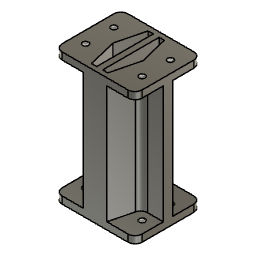
0812_arm_short v2 (Autodesk Fusion 360 design; units mm, degrees)
Autodesk Fusion 360 part; units mm, degrees
sketch "스케치1" plane through (0, 0, 0) normal (0, 0, 1) x (1, 0, 0)
  line L0 (-17, 14) -> (17, 14)
  line L1 (17, 14) -> (17, -14)
  line L2 (17, -14) -> (-17, -14)
  line L3 (-17, -14) -> (-17, 14)
  line L4 (0, 14) -> (0, -14) construction
  line L5 (-12, 6) -> (12, 6) construction
  line L6 (12, 6) -> (12, -6) construction
  line L7 (12, -6) -> (-12, -6) construction
  line L8 (-12, -6) -> (-12, 6) construction
  line L9 (0, 6) -> (0, -6) construction
  circle A0 centre (-12, 6) radius 1.5
  circle A1 centre (12, 6) radius 1.5
  circle A2 centre (-12, -6) radius 1.5
  circle A3 centre (12, -6) radius 1.5
  line L10 (-5, 14) -> (5, 14)
  line L11 (5, 14) -> (5, -14) construction
  line L12 (5, -14) -> (-5, -14)
  line L13 (-5, -14) -> (-5, 14) construction
  line L14 (-17, 2) -> (17, 2) construction
  line L15 (17, 2) -> (17, -2)
  line L16 (17, -2) -> (-17, -2) construction
  line L17 (-17, -2) -> (-17, 2)
  line L18 (0, 2) -> (0, -2) construction
  line L19 (0, 14) -> (0, -14) construction
  line L20 (-5, 14) -> (-8, 2)
  line L21 (5, 14) -> (8, 2)
  line L22 (-8, -2) -> (-5, -14)
  line L23 (8, -2) -> (5, -14)
  line L24 (-17, 2) -> (-8, 2)
  line L25 (8, 2) -> (17, 2)
  line L26 (8, -2) -> (17, -2)
  line L27 (-17, -2) -> (-8, -2)
  line L28 (-3.4384, 12) -> (3.4384, 12)
  line L29 (3.4384, 12) -> (6.4384, 0)
  line L30 (6.4384, 0) -> (3.4384, -12)
  line L31 (3.4384, -12) -> (-3.4384, -12)
  line L32 (-3.4384, -12) -> (-6.4384, 0)
  line L33 (-6.4384, 0) -> (-3.4384, 12)
  line L34 (0, 12) -> (0, -12) construction
  line L35 (-6.4384, 0) -> (6.4384, 0) construction
  line L36 (-1.25, 14) -> (1.25, 14)
  line L37 (1.25, 14) -> (1.25, -14)
  line L38 (1.25, -14) -> (-1.25, -14)
  line L39 (-1.25, -14) -> (-1.25, 14)
  line L40 (0, 14) -> (0, -14) construction
  point P0 (0, 14)
  point P1 (0, -14)
  point P2 (0, 6)
  point P3 (0, -6)
  point P4 (0, 2)
  point P5 (0, -2)
  point P6 (0, 14)
  point P7 (0, -14)
  point P8 (-8, 2)
  point P9 (-8, -2)
  point P10 (8, 2)
  point P11 (8, -2)
  point P12 (-17, 2)
  point P13 (-17, -2)
  point P14 (17, -2)
  point P15 (17, 2)
  point P16 (0, 12)
  point P17 (0, -12)
  point P18 (0, 14)
  point P19 (0, -14)
  point P20 (-1.25, 12)
  point P21 (-1.25, 12)
  point P22 (1.25, 12)
  point P23 (1.25, 12)
  point P24 (-1.25, -12)
  point P25 (-1.25, -12)
  point P26 (1.25, -12)
  point P27 (1.25, -12)
  dimension "d1" = 34
  dimension "d2" = 28
  dimension "d3" = 24
  dimension "d4" = 12
  dimension "d5" = 3
  dimension "d6" = 3
  dimension "d7" = 3
  dimension "d8" = 3
  dimension "d11" = 10
  dimension "d12" = 28
  dimension "d13" = 34
  dimension "d14" = 4
  dimension "d15" = 9
  dimension "d16" = 9
  dimension "d17" = 9
  dimension "d18" = 9
  dimension "d19" = 2
  dimension "d20" = 2
  dimension "d21" = 2
  dimension "d22" = 2.5
  dimension "d23" = 28
  constraint horizontal L0
  constraint vertical L1
  constraint horizontal L2
  constraint vertical L3
  constraint midpoint L0 P18
  constraint midpoint L2 P19
  constraint coincident P18 P6
  constraint coincident P19 P7
  constraint midpoint L4 origin
  constraint horizontal L5
  constraint vertical L6
  constraint horizontal L7
  constraint vertical L8
  constraint midpoint L5 P2
  constraint midpoint L7 P3
  constraint coincident P2 L9.start
  constraint coincident P3 L9.end
  constraint midpoint L9 origin
  constraint coincident L5.start L8.end
  constraint coincident L5.end L6.start
  constraint coincident L7.end L8.start
  constraint coincident L6.end L7.start
  constraint horizontal L10
  constraint vertical L11
  constraint horizontal L12
  constraint vertical L13
  constraint horizontal L14
  constraint vertical L15
  constraint horizontal L16
  constraint vertical L17
  constraint midpoint L14 P4
  constraint midpoint L16 P5
  constraint coincident P4 L18.start
  constraint coincident P5 L18.end
  constraint midpoint L18 origin
  constraint midpoint L10 P18
  constraint midpoint L12 P19
  constraint midpoint L19 origin
  constraint coincident L14 P8
  constraint coincident L16 P9
  constraint coincident L14 P10
  constraint coincident L16 P11
  constraint coincident P12 L14.start
  constraint coincident P13 L16.end
  constraint coincident P14 L15.end
  constraint coincident P15 L14.end
  constraint coincident P8 L20.end
  constraint coincident P10 L21.end
  constraint coincident P9 L22.start
  constraint coincident P11 L23.start
  constraint horizontal L28
  constraint parallel L28 L31
  constraint midpoint L28 P16
  constraint midpoint L31 P17
  constraint coincident P16 L34.start
  constraint coincident P17 L34.end
  constraint midpoint L34 origin
  constraint perpendicular L28 L34
  constraint coincident L29 L30.start
  constraint midpoint L35 origin
  constraint perpendicular L34 L35
  constraint parallel L21 L29
  constraint parallel L23 L30
  constraint horizontal L36
  constraint vertical L37
  constraint horizontal L38
  constraint vertical L39
  constraint midpoint L36 P18
  constraint midpoint L38 P19
  constraint midpoint L40 origin
  constraint coincident L28 P21
  constraint coincident L39 P21
  constraint coincident P21 P20
  constraint coincident L28 P23
  constraint coincident L37 P23
  constraint coincident P23 P22
  constraint coincident L31 P25
  constraint coincident L39 P25
  constraint coincident L31 P27
  constraint coincident L37 P27
  constraint coincident P25 P24
  constraint coincident P27 P26
  measures "d1" distance of L0.start L0.end
  measures "d2" distance of L0.start L2.end
  measures "d3" distance of L5.start L5.end
  measures "d4" distance of L5.start L7.end
  measures "d5" diameter of A0
  measures "d6" diameter of A1
  measures "d7" diameter of A2
  measures "d8" diameter of A3
  measures "d11" distance of L10.start L10.end
  measures "d12" distance of L10.start L12.end
  measures "d13" distance of P12 P15
  measures "d14" distance of P12 P13
  measures "d15" distance of P8 P12
  measures "d16" distance of P9 P13
  measures "d17" distance of P10 P15
  measures "d18" distance of P11 P14
  measures "d19" distance of L10 L28
  measures "d20" distance of L21 L29
  measures "d21" distance of L23 L30
  measures "d22" distance of L36.start L36.end
  measures "d23" distance of L36.start L38.end
extrude "돌출2" add sketch "스케치1" along normal blind 56 contours L0 L2 L3 L10 L12 L17 L20 L22 L24 L27 L28 L31 L32 L33 L39 | L0 L10 L28 L36 L37 L39 | L0 L1 L2 L10 L12 L15 L21 L23 L25 L26 L28 L29 L30 L31 L37 | L28 L31 L37 L39 | L2 L12 L31 L37 L38 L39
extrude "돌출3" add sketch "스케치1" along normal blind 3 contours L0 L3 L20 L24 | L2 L3 L22 L27 | L0 L1 L21 L25 | L1 L2 L23 L26
extrude "돌출4" add sketch "스케치1" along normal blind 3 from surface at 53 contours L0 L3 L20 L24 | L2 L3 L22 L27 | L0 L1 L21 L25 | L1 L2 L23 L26
extrude "돌출5" add sketch "스케치1" along normal blind 3 contours L28 L31 L32 L33 L39 | L28 L29 L30 L31 L37
thread "스레드1" "ISO Metric profile 3.0 M3x0.5 6H" major diameter 3.086 minor diameter 2.529 pitch 0.5 angle 60 resizes the face on face at (-10.5019, 5.9252, 55)
thread "스레드2" "ISO Metric profile 3.0 M3x0.5 6H" major diameter 3.086 minor diameter 2.529 pitch 0.5 angle 60 resizes the face on face at (-10.5019, -6.0748, 55)
thread "스레드3" "ISO Metric profile 3.0 M3x0.5 6H" major diameter 3.086 minor diameter 2.529 pitch 0.5 angle 60 resizes the face on face at (13.4981, 5.9252, 55)
thread "스레드4" "ISO Metric profile 3.0 M3x0.5 6H" major diameter 3.086 minor diameter 2.529 pitch 0.5 angle 60 resizes the face on face at (13.4981, -6.0748, 55)
thread "스레드5" "ISO Metric profile 3.0 M3x0.5 6H" major diameter 3.086 minor diameter 2.529 pitch 0.5 angle 60 resizes the face on face at (13.4981, -6.0748, 2)
thread "스레드6" "ISO Metric profile 3.0 M3x0.5 6H" major diameter 3.086 minor diameter 2.529 pitch 0.5 angle 60 resizes the face on face at (-10.5019, -6.0748, 2)
thread "스레드7" "ISO Metric profile 3.0 M3x0.5 6H" major diameter 3.086 minor diameter 2.529 pitch 0.5 angle 60 resizes the face on face at (13.4981, 5.9252, 2)
thread "스레드8" "ISO Metric profile 3.0 M3x0.5 6H" major diameter 3.086 minor diameter 2.529 pitch 0.5 angle 60 resizes the face on face at (-10.5019, 5.9252, 2)
fillet "모깎기1" radius 3 8 edges at (17, 14, 54.5) (-17, 14, 54.5) (-17, -14, 54.5) (17, -14, 54.5) (-17, -14, 1.5) (17, -14, 1.5) (17, 14, 1.5) (-17, 14, 1.5)
fillet "모깎기2" radius 3 4 edges at (-8, 2, 28) (-8, -2, 28) (8, -2, 28) (8, 2, 28)
extrude "돌출1" [rolled back] along distance 3 taper angle 0
sketch "스케치2" plane through (0, 0, 3) normal (0, 0, 1) x (-1, 0, 0)
  circle A0 centre (12, -6) radius 1.5
  circle A1 centre (12, 6) radius 1.5
  circle A2 centre (-12, -6) radius 1.5
  circle A3 centre (-12, 6) radius 1.5
  line L0 (19, 12) -> (-19, 12)
  line L1 (-19, 12) -> (-19, -12)
  line L2 (-19, -12) -> (19, -12)
  line L3 (19, -12) -> (19, 12)
